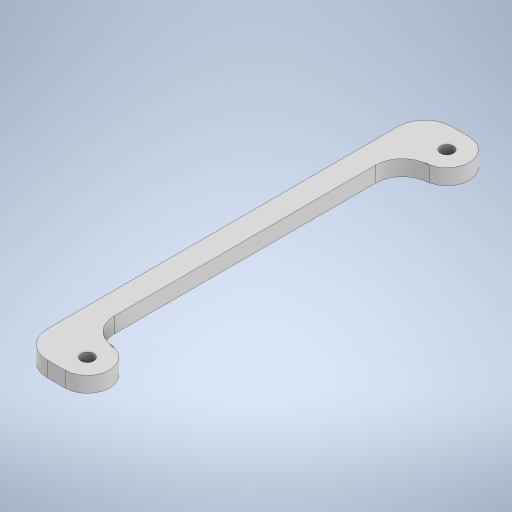
# Autodesk Inventor part: sidemount
Saved by Autodesk Inventor 2023 (Build 270158000, 158)
## iProperties
Created: 2022-12-04
Part Number: sidemount
Material: Generic
Document SubType Name: Modeling
Designer: user
Density: 1 g/cm^3
Appearance: Default
Author: user
Autodesk Inventor part; units mm, degrees
ref_plane "YZ Plane" through (0, 0, 0) normal (1, 0, 0) x (0, 1, 0)
ref_plane "XZ Plane" through (0, 0, 0) normal (0, 1, 0) x (-1, 0, 0)
ref_plane "XY Plane" through (0, 0, 0) normal (0, 0, 1) x (1, 0, 0)
sketch "Sketch1" plane through (0, 0, 0) normal (0, 1, 0) x (-1, 0, 0)
  circle A0 centre (0, 0) radius 1.4732
  circle A1 centre (0, -80.9498) radius 1.4732
  circle A2 centre (0, 0) radius 5.0165
  circle A3 centre (0, -80.9498) radius 5.0165
  line L0 (0, 5.0165) -> (4.033, 5.0165)
  line L1 (4.033, -85.9663) -> (0, -85.9663)
  line L2 (10.033, -79.9663) -> (10.033, -0.9835)
  line L3 (0, -5.0165) -> (-0.9835, -5.0165)
  line L4 (5.0165, -11.0165) -> (5.0165, -69.9333)
  line L5 (-0.9835, -75.9333) -> (0, -75.9333)
  arc A4 (10.033, -0.9835) -> (4.033, 5.0165) centre (4.033, -0.9835) ccw
  arc A5 (4.033, -85.9663) -> (10.033, -79.9663) centre (4.033, -79.9663) ccw
  arc A6 (5.0165, -11.0165) -> (-0.9835, -5.0165) centre (-0.9835, -11.0165) ccw
  arc A7 (-0.9835, -75.9333) -> (5.0165, -69.9333) centre (-0.9835, -69.9333) ccw
  point P0 (10.033, 5.0165)
  dimension "d0" = 2.9464
  dimension "d2" = 2.9464
  dimension "d3" = 10.033
  dimension "d4" = 10.033
  dimension "d7" = 80.9498
  dimension "d8" = 10.033
  dimension "d9" = 6
  dimension "d10" = 6
  dimension "d11" = 6
  dimension "d12" = 6
  constraints: 12 end point, 12 point on circle, 11 tangent, 8 centre point, 3 coincident, 2 perpendicular, 2 point on line, 1 horizontal
  measures "d0" diameter of A0
  measures "d2" diameter of A1
  measures "d3" diameter of A2
  measures "d4" diameter of A3
  measures "d7" distance of A2.centre A3.centre
  measures "d8" distance of L0.start point (10.033, 5.017)
  measures "d9" radius of A4
  measures "d10" radius of A5
  measures "d11" radius of A6
  measures "d12" radius of A7
extrude "Extrusion1" add sketch "Sketch1" along normal blind 3.5
body "Solid1"
